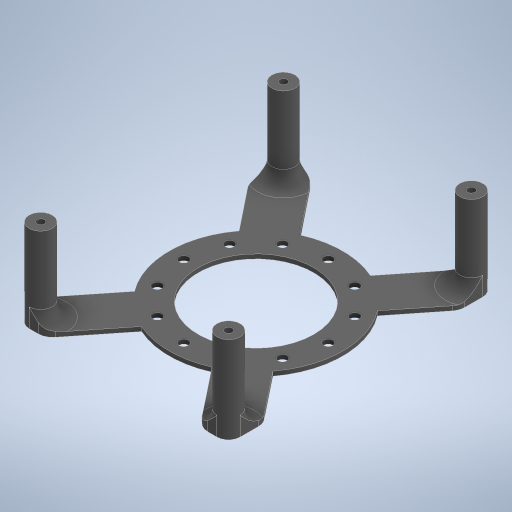
# Autodesk Inventor part: board_base_connect
Saved by Autodesk Inventor 2024.1 (Build 281209000, 209)
## iProperties
Created: 2024-08-02
Part Number: board_base_connect
Material: 一般
Document SubType Name: Modeling
Designer: hibik
Density: 1 g/cm^3
Appearance: 既定
Author: hibik
Autodesk Inventor part; units mm, degrees
ref_plane "YZ Plane" through (0, 0, 0) normal (1, 0, 0) x (0, 1, 0)
ref_plane "XZ Plane" through (0, 0, 0) normal (0, 1, 0) x (-1, 0, 0)
ref_plane "XY Plane" through (0, 0, 0) normal (0, 0, 1) x (1, 0, 0)
sketch "スケッチ1" plane through (0, 0, 0) normal (0, 1, 0) x (-1, 0, 0)
  line L0 (-32.5, -42) -> (32.5, -42) construction
  line L1 (32.5, -42) -> (32.5, 42) construction
  line L2 (32.5, 42) -> (-32.5, 42) construction
  line L3 (-32.5, 42) -> (-32.5, -42) construction
  line L4 (-32.5, -42) -> (32.5, 42) construction
  line L5 (32.5, -42) -> (-32.5, 42) construction
  circle A0 centre (32.5, 42) radius 4
  circle A1 centre (32.5, -42) radius 4
  circle A2 centre (-32.5, -42) radius 4
  circle A3 centre (-32.5, 42) radius 4
  circle A4 centre (32.5, 42) radius 1.3
  circle A5 centre (32.5, -42) radius 1.3
  circle A6 centre (-32.5, 42) radius 1.3
  circle A7 centre (-32.5, -42) radius 1.3
  point P0 (0, 0)
  dimension "d0" = 65
  dimension "d1" = 84
  dimension "d2" = 8
  dimension "d4" = 2.6
  constraints: 12 end point, 8 centre point, 8 coincident, 6 equal radius, 2 midpoint, 2 parallel, 1 horizontal, 1 perpendicular
  measures "d0" distance of L2.end L1.end
  measures "d1" distance of L1.end L0.end
  measures "d2" diameter of A0
  measures "d4" diameter of A4
extrude "押し出し1" add sketch "スケッチ1" along normal blind 30
sketch "スケッチ2" plane through (32.5, 0, 42) normal (0, -1, 0) x (1, 0, 0)
  circle A0 centre (-32.5, -42) radius 20
  circle A1 centre (-32.5, -42) radius 30
  circle A2 centre (-32.5, -17) radius 1.6
  line L0 (-32.5, -42) -> (-32.5, -12) construction
  line L1 (-32.5, -22) -> (-32.5, -12)
  circle A3 centre (-45, -20.3494) radius 1.6
  circle A4 centre (-54.1506, -29.5) radius 1.6
  circle A5 centre (-57.5, -42) radius 1.6
  circle A6 centre (-54.1506, -54.5) radius 1.6
  circle A7 centre (-45, -63.6506) radius 1.6
  circle A8 centre (-32.5, -67) radius 1.6
  circle A9 centre (-20, -63.6506) radius 1.6
  circle A10 centre (-10.8494, -54.5) radius 1.6
  circle A11 centre (-7.5, -42) radius 1.6
  circle A12 centre (-10.8494, -29.5) radius 1.6
  circle A13 centre (-20, -20.3494) radius 1.6
  line L2 (-69, 4) -> (4, 4)
  line L3 (4, 4) -> (4, -88)
  line L4 (4, -88) -> (-69, -88)
  line L5 (-69, -88) -> (-69, 4)
  circle A14 centre (0, 0) radius 4 projected
  circle A15 centre (0, -84) radius 4 projected
  circle A16 centre (-65, -84) radius 4 projected
  circle A17 centre (-65, 0) radius 4 projected
  line L6 (9.8752, -0.6618) -> (-63.1248, -92.6618)
  line L7 (-63.1248, -92.6618) -> (-74.8752, -83.3382)
  line L8 (-74.8752, -83.3382) -> (-1.8752, 8.6618)
  line L9 (-1.8752, 8.6618) -> (9.8752, -0.6618)
  line L10 (9.8752, -0.6618) -> (-74.8752, -83.3382) construction
  line L11 (-63.1248, -92.6618) -> (-1.8752, 8.6618) construction
  line L12 (9.8752, -83.3382) -> (-63.1248, 8.6618)
  line L13 (-63.1248, 8.6618) -> (-74.8752, -0.6618)
  line L14 (-74.8752, -0.6618) -> (9.8752, -83.3382) construction
  line L15 (-30.3791, -45.5085) -> (-63.1248, 8.6618) construction
  line L16 (-74.8752, -0.6618) -> (-1.8752, -92.6618)
  line L17 (-1.8752, -92.6618) -> (9.8752, -83.3382)
  line L18 (-1.8752, -92.6618) -> (-63.1248, 8.6618) construction
  point P0 (-69, 0)
  point P1 (-69, -84)
  point P2 (-65, -88)
  point P3 (0, -88)
  point P4 (4, -84)
  point P5 (4, 0)
  point P6 (0, 4)
  point P7 (-65, 4)
  point P8 (-20.32, -14.5838)
  point P9 (-44.68, -14.5838)
  point P10 (-59.4258, 4)
  point P11 (-56.4303, -60.0926)
  point P12 (-69, -75.9339)
  point P13 (-59.4258, -88)
  point P14 (-44.68, -69.4162)
  point P15 (4, -75.9339)
  point P16 (-8.5697, -60.0926)
  point P17 (-8.5697, -23.9074)
  point P18 (4, -8.0661)
  point P19 (-5.5742, 4)
  point P20 (-61.3653, -1.6701)
  point P21 (-66.5796, 3.6749)
  point P22 (4, 4)
  point P23 (4, 4)
  point P24 (-22.9258, -42)
  point P25 (-32.5, -29.9339)
  point P26 (-15.1005, -51.862)
  point P27 (-38.1491, -61.1856)
  point P28 (-49.8995, -51.862)
  point P29 (-38.1491, -22.8144)
  point P30 (-26.8509, -22.8144)
  point P31 (-15.1005, -32.138)
  point P32 (-32.5, -42)
  point P33 (-32.5, -42)
  point P34 (-69, -8.0661)
  point P35 (-56.4303, -23.9074)
  point P36 (-20.32, -69.4162)
  point P37 (-5.5742, -88)
  dimension "d7" = 40
  dimension "d8" = 60
  dimension "d9" = 3.2
  dimension "d12" = 360
  dimension "d17" = 15
  constraints: 38 end point, 12 centre point, 10 midpoint, 5 perpendicular, 4 parallel, 4 tangent, 3 point on line, 2 coincident, 1 collinear, 1 equal length, 1 horizontal, 1 vertical, 31 other
  measures "d9" diameter of A2
  measures "d17" distance between parallel lines of L8 L6
extrude "押し出し2" add sketch "スケッチ2" against normal blind 1.5 contours A0 L6 A1 L12 | A0 L8 A1 L6 | L12 A1 L16 A0 | A0 L1 A2 A1 L8 | A1 L8 L2 A14 L3 L6 | L16 A1 L6 A0 | L12 L3 A15 L4 L16 A1 | A0 L12 A1 L1 A2 | L6 A1 L8 A0 | A0 L16 A1 L12 | A14 L2 L3 | A14 | L8 A1 L16 A0 | L6 L4 A16 L5 L8 A1 | A15 | L3 L4 A15 | A1 L16 L5 A17 L2 L12 | A17 L5 L2 | A17 | L4 L5 A16 | A16
fillet "フィレット2" radius 4 4 edges at (-36.5, 0.75, 46) (36.5, 0.75, 46) (36.5, 0.75, -46) (-36.5, 0.75, -46)
fillet "フィレット3" radius 5 14 edges at (-29.6716, 1.5, -39.1716) (32.5, 1.5, -38) (29.6716, 1.5, -44.8284) (-29.6716, 1.5, 39.1716) (29.6716, 1.5, 44.8284) (32.5, 1.5, 38) (36.5, 0.75, 33.9339) (26.9258, 0.75, -46) (-36.5, 0.75, -33.9339) (-26.9258, 0.75, 46) (-36.5, 0.75, 33.9339) (-26.9258, 0.75, -46) (36.5, 0.75, -33.9339) (26.9258, 0.75, 46)
